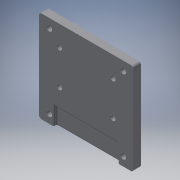
# Autodesk Inventor part: крепеж камеры
Saved by Autodesk Inventor 2019.1 (Build 231200000, 200)
## iProperties
Created: 2018-09-16
Part Number: крепеж камеры
Material: Типовые
Document SubType Name: Modeling
Designer: Олег
Density: 1 g/cm^3
Appearance: По умолчанию
Author: Олег
Autodesk Inventor part; units mm, degrees
ref_plane "YZ Plane" through (0, 0, 0) normal (1, 0, 0) x (0, 1, 0)
ref_plane "XZ Plane" through (0, 0, 0) normal (0, 1, 0) x (-1, 0, 0)
ref_plane "XY Plane" through (0, 0, 0) normal (0, 0, 1) x (1, 0, 0)
sketch "Эскиз1" plane through (0, 0, 0) normal (0, 0, 1) x (1, 0, 0)
  line L0 (18.5, -18) -> (-18.5, -18)
  line L1 (-18.5, -18) -> (-18.5, 18)
  line L2 (-18.5, 18) -> (18.5, 18)
  line L3 (18.5, 18) -> (18.5, -18)
  line L4 (18.5, -18) -> (-18.5, 18) construction
  line L5 (-18.5, -18) -> (18.5, 18) construction
  line L6 (-14.5, -14.5) -> (14.5, -14.5) construction
  line L7 (14.5, -14.5) -> (14.5, 14.5) construction
  line L8 (14.5, 14.5) -> (-14.5, 14.5) construction
  line L9 (-14.5, 14.5) -> (-14.5, -14.5) construction
  line L10 (-14.5, -14.5) -> (14.5, 14.5) construction
  line L11 (14.5, -14.5) -> (-14.5, 14.5) construction
  circle A0 centre (-14.5, 14.5) radius 1.1
  circle A1 centre (14.5, 14.5) radius 1.1
  circle A2 centre (-14.5, -14.5) radius 1.1
  circle A3 centre (14.5, -14.5) radius 1.1
  point P0 (0, 0)
  dimension "d0" = 37
  dimension "d1" = 36
  dimension "d2" = 29
  dimension "d3" = 29
  dimension "d4" = 2.2
  dimension "d7" = 29
  dimension "d10" = 29
  constraints: 24 end point, 4 centre point, 4 midpoint, 4 parallel, 3 horizontal, 2 perpendicular, 1 coincident, 1 vertical, 6 other
  measures "d0" distance of L1.end L2.end
  measures "d1" distance of L0.end L1.end
  measures "d2" distance of L8.end L7.end
  measures "d3" distance of L7.end L6.end
  measures "d4" diameter of A0
  measures "d7" distance of A0.centre A1.centre
  measures "d10" distance of A0.centre A2.centre
extrude "Выдавливание1" add sketch "Эскиз1" along normal blind 3
fillet "Сопряжение1" radius 1 4 edges at (-18.5, 18, 1.5) (18.5, 18, 1.5) (18.5, -18, 1.5) (-18.5, -18, 1.5)
sketch "Эскиз2" plane through (0, 0, 3) normal (0, 0, 1) x (1, 0, 0)
  circle A0 centre (10.5, -3.5) radius 1 projected
  circle A1 centre (10.5, 10) radius 1 projected
  circle A2 centre (-10.5, 10) radius 1 projected
  circle A3 centre (-10.5, -3.5) radius 1 projected
  point P0 (0, 0)
extrude "Выдавливание2" cut sketch "Эскиз2" against normal blind 3
sketch "Эскиз3" plane through (0, 0, 0) normal (0, 0, -1) x (-1, 0, 0)
  circle A0 centre (10.5, -3.5) radius 1 projected
  circle A1 centre (-10.5, -3.5) radius 1 projected
  circle A2 centre (10.5, 10) radius 1 projected
  circle A3 centre (-10.5, 10) radius 1 projected
  circle A4 centre (10.5, -3.5) radius 2
  circle A5 centre (-10.5, -3.5) radius 2
  circle A6 centre (-10.5, 10) radius 2
  circle A7 centre (10.5, 10) radius 2
  point P0 (0, 0)
  dimension "d18" = 1
  dimension "d19" = 1
  dimension "d20" = 1
  dimension "d21" = 1
  constraints: 4 centre point
  measures "d18" radial gap between concentric circles of A0 A4
  measures "d19" radial gap between concentric circles of A1 A5
  measures "d20" radial gap between concentric circles of A3 A6
  measures "d21" radial gap between concentric circles of A2 A7
extrude "Выдавливание3" cut sketch "Эскиз3" against normal blind 2
sketch "Эскиз4" plane through (0, 0, 3) normal (0, 0, 1) x (1, 0, 0)
  line L0 (-12.5, -12) -> (12.5, -12) construction
  line L1 (12.5, -12) -> (12.5, -18) construction
  line L2 (-17.5, -18) -> (17.5, -18) construction
  line L3 (-12.5, -12) -> (-12.5, -18) construction
  line L4 (12.5, -18) -> (-12.5, -18)
  line L5 (-12.5, -18) -> (-12.5, -11)
  line L6 (-12.5, -11) -> (12.5, -11)
  line L7 (12.5, -11) -> (12.5, -18)
  point P0 (0, 0)
  dimension "d24" = 7
  constraints: 12 end point, 3 parallel, 3 point on line, 1 horizontal, 1 perpendicular, 1 vertical
  measures "d24" distance between parallel lines of L2 L6
extrude "Выдавливание4" cut sketch "Эскиз4" against normal blind 1
fillet "Сопряжение2" radius 0.5 9 edges at (0, -11, 3) (0, -11, 2) (0, -18, 2) (12.5, -18, 2.5) (12.5, -14.5, 2) (-12.5, -18, 2.5) (-12.5, -14.5, 2) (12.5, -14.5, 3) (-12.5, -14.5, 3)
